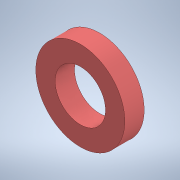
# Autodesk Inventor part: bearing
Saved by Autodesk Inventor 2020.1 (Build 241239000, 239)
## iProperties
Created: 2020-01-18
Part Number: bearing
Material: Generic
Document SubType Name: Modeling
Designer: Ali
Density: 1 g/cm^3
Appearance: Default
Author: Ali
Autodesk Inventor part; units mm, degrees
ref_plane "YZ Plane" through (0, 0, 0) normal (1, 0, 0) x (0, 1, 0)
ref_plane "XZ Plane" through (0, 0, 0) normal (0, 1, 0) x (-1, 0, 0)
ref_plane "XY Plane" through (0, 0, 0) normal (0, 0, 1) x (1, 0, 0)
sketch "Sketch1" plane through (0, 0, 0) normal (0, 0, 1) x (1, 0, 0)
  circle A0 centre (0, 0) radius 1.3
  circle A1 centre (0, 0) radius 2.3
  dimension "d0" = 2.6
  dimension "d1" = 1
  constraints: 2 centre point, 2 coincident
  measures "d0" diameter of A0
  measures "d1" radial gap between concentric circles of A0 A1
extrude "Extrusion1" add sketch "Sketch1" along normal blind 1
equation "\"d0\" = IG_shaftDiameter + W_holesClearance"
equation "\"d1\" = B_bearingThickness"
equation "\"d2\" = W_wallThickness"
equation "\"Wheel_Related_W_\" = 0"
equation "\"W_innerDiameter\" = 35"
equation "\"W_wallThickness\" = 1"
equation "\"W_holesClearance\" = 0.1"
equation "\"W_outerGearHoleDiameter\" = 1.7"
equation "\"W_innerGearHoleDiameter\" = 4.7"
equation "\"TempSpotReserved7\" = 0"
equation "\"TempSpotReserved8\" = 0"
equation "\"TempSpotReserved9\" = 0"
equation "\"TempSpotReserved10\" = 0"
equation "\"Inner_Gear_Related_IG_\" = 0"
equation "\"IG_shaftDiameter\" = 2.5"
equation "\"IG_shaftLength\" = 15"
equation "\"IG_gearThickness\" = 1"
equation "\"TempSpotReserved16\" = 0"
equation "\"TempSpotReserved17\" = 0"
equation "\"TempSpotReserved18\" = 0"
equation "\"TempSpotReserved19\" = 0"
equation "\"TempSpotReserved20\" = 0"
equation "\"Outer_Gear_Related_OG_\" = 0"
equation "\"OG_shaftDiameter\" = 1.5"
equation "\"OG_gearThickness\" = 2"
equation "\"TempSpotReserved27\" = 0"
equation "\"TempSpotReserved28\" = 0"
equation "\"TempSpotReserved29\" = 0"
equation "\"TempSpotReserved30\" = 0"
equation "\"Leg_Extensions_Related_LE_\" = 0"
equation "\"LE_baseDiameter\" = 2"
equation "\"LE_maxLength\" = 10.64459"
equation "\"LE_thickness\" = 2"
equation "\"TempSpotReserved47\" = 0"
equation "\"B_bearingThickness\" = 1"
equation "\"TempSpotReserved50\" = 0"
equation "\"TempSpotReserved43\" = 0"
equation "\"TempSpotReserved45\" = 0"
equation "\"Thisisatest\" = 25.4"
equation "\"TempSpotReserved48\" = 0"
equation "\"TempSpotReserved46\" = 0"
equation "\"TempSpotReserved44\" = 0"
equation "\"TempSpotReserved49\" = 0"
equation "\"TempSpotReserved35\" = 0"
equation "\"TempSpotReserved39\" = 0"
equation "\"TempSpotReserved38\" = 0"
equation "\"TempSpotReserved37\" = 0"
equation "\"LE_offsetAboveOuterGear\" = 0"
equation "\"TempSpotReserved36\" = 0"
equation "\"TempSpotReserved40\" = 0"
equation "\"Bearing_Related_B_\" = 0"
equation "\"TempSpotReserved42\" = 0"
equation "\"OG_skirtOffset\" = 1"
equation "\"OG_skirtThickness\" = 1"
equation "\"IG_skirtThickness\" = 0.5"
equation "\"IG_skirtOffset\" = 1.5"
body "Solid1"
